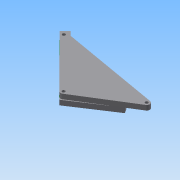
# Autodesk Inventor part: 1-4
Saved by Autodesk Inventor 2015 (Build 190159000, 159)
## iProperties
Created: 2018-05-07
Part Number: 1-4
Material: 一般
Document SubType Name: Modeling
Designer: 王博聖
Density: 1 g/cm^3
Appearance: 預設
Author: 王博聖
Autodesk Inventor part; units mm, degrees
ref_plane "YZ Plane" through (0, 0, 0) normal (1, 0, 0) x (0, 1, 0)
ref_plane "XZ Plane" through (0, 0, 0) normal (0, 1, 0) x (-1, 0, 0)
sketch "草圖1" plane through (0, 0, 0) normal (0, 0, 1) x (1, 0, 0)
  line L0 (0, 0) -> (-20.3496, 20.4644)
  line L1 (-20.3496, 20.4644) -> (21.2832, 13.2109)
  line L2 (21.2832, 13.2109) -> (0, 0)
  line L3 (0, 0) -> (-20.3496, 20.4644) construction
  line L4 (0.8864, 0.8814) -> (-19.4632, 21.3458)
  line L5 (-21.236, 19.583) -> (-0.8864, -0.8814)
  arc A0 (-0.8864, -0.8814) -> (0.8864, 0.8814) centre (0, 0) ccw
  arc A1 (-19.4632, 21.3458) -> (-21.236, 19.583) centre (-20.3496, 20.4644) ccw
  line L6 (-20.3496, 20.4644) -> (21.2832, 13.2109) construction
  line L7 (-20.5642, 19.233) -> (21.0687, 11.9794)
  line L8 (21.4978, 14.4423) -> (-20.1351, 21.6959)
  arc A2 (-20.1351, 21.6959) -> (-20.5642, 19.233) centre (-20.3496, 20.4644) ccw
  arc A3 (21.0687, 11.9794) -> (21.4978, 14.4423) centre (21.2832, 13.2109) ccw
  line L9 (21.2832, 13.2109) -> (0, 0) construction
  line L10 (20.624, 14.2729) -> (-0.6592, 1.062)
  line L11 (0.6592, -1.062) -> (21.9425, 12.1488)
  arc A4 (21.9425, 12.1488) -> (20.624, 14.2729) centre (21.2832, 13.2109) ccw
  arc A5 (-0.6592, 1.062) -> (0.6592, -1.062) centre (0, 0) ccw
  point P0 (-10.1748, 10.2322)
  point P1 (0.4668, 16.8376)
  point P2 (10.6416, 6.6054)
  dimension "d0" = 28.86
  dimension "d1" = 42.26
  dimension "d2" = 25.05
  dimension "d3" = 2.5
  dimension "d4" = 2.5
  dimension "d5" = 2.5
  constraints: 30 end point, 12 point on circle, 12 tangent, 6 centre point, 4 equal length, 3 midpoint, 1 concentric
  measures "d0" distance of L0.start L0.end
  measures "d1" distance of L0.end L1.end
  measures "d2" distance of L1.end L0.start
  measures "d3" diameter of A1
  measures "d4" diameter of A3
  measures "d5" diameter of A5
extrude "擠出1" add sketch "草圖1" along normal blind 2 contours L2 A0 A5 L0 | L0 A5 L10 L4 A0 L2 | A5 L5 A2 L7 L0 | L0 L7 L4 L10 A5 | A0 L4 L10 L7 L2 | L2 L7 A3 L11 A0 | L7 A2 A1 L4 L1 L0 | L0 L1 L4 L7 | L7 L10 L1 L2 | L2 L1 L10 A4 A3 L7 | L4 L1 L10 L7 | L4 A1 L8 A4 L10 L1
sketch "草圖2" plane through (0, 0, 2) normal (0, 0, 1) x (1, 0, 0)
  arc A0 (21.9425, 12.1488) -> (21.4978, 14.4423) centre (21.2832, 13.2109) ccw construction
  arc A1 (-20.1351, 21.6959) -> (-21.236, 19.583) centre (-20.3496, 20.4644) ccw construction
  arc A2 (-0.8864, -0.8814) -> (0.6592, -1.062) centre (0, 0) ccw construction
  circle A3 centre (0, 0) radius 0.625
  circle A4 centre (21.2832, 13.2109) radius 0.625
  circle A5 centre (-20.3496, 20.4644) radius 0.625
  dimension "d8" = 1.25
  dimension "d9" = 1.25
  dimension "d10" = 1.25
  constraints: 3 centre point, 3 coincident
  measures "d8" diameter of A3
  measures "d9" diameter of A4
  measures "d10" diameter of A5
extrude "擠出2" cut sketch "草圖2" against normal blind 2
sketch "草圖3" plane through (0, 0, 0) normal (0, 0, -1) x (-1, 0, 0)
  circle A0 centre (20.3496, 20.4644) radius 0.625 projected
  line L0 (21.236, 19.583) -> (0.8864, -0.8814) projected
  arc A1 (21.236, 19.583) -> (20.1351, 21.6959) centre (20.3496, 20.4644) ccw projected
  line L1 (-21.4978, 14.4423) -> (20.1351, 21.6959) projected
  line L2 (-9.4658, 16.5386) -> (7.2751, 5.5434)
  constraints: 2 end point, 2 point on line
extrude "擠出3" add sketch "草圖3" along normal blind 8
extrude "擠出4" cut sketch "草圖3" along normal blind 6
sketch "草圖4" plane through (-7.2751, 5.5434, -8) normal (0.5489701, -0.835842, 0) x (0.835842, 0.5489701, 0)
  line L0 (20.0288, 0) -> (0, 0)
  line L1 (0, 0) -> (0, 8)
  line L2 (0, 8) -> (20.0288, 8)
  line L3 (20.0288, 8) -> (20.0288, 0)
  point P0 (3.0377, 8)
  constraints: 8 end point, 2 parallel, 1 horizontal, 1 perpendicular
extrude "擠出5" add sketch "草圖4" along normal blind 2
sketch "草圖5" plane through (-7.2751, 5.5434, -8) normal (-0.5489701, 0.835842, 0) x (0.835842, 0.5489701, 0)
  line L0 (0, -8) -> (0, -2) projected
  line L1 (8, -2) -> (-8, -2)
  line L2 (-8, -2) -> (-8, -8)
  line L3 (-8, -8) -> (8, -8)
  line L4 (8, -8) -> (8, -2)
  line L5 (8, -2) -> (-8, -8) construction
  line L6 (-8, -2) -> (8, -8) construction
  point P0 (3.0377, -8)
  point P1 (0, -5)
  dimension "d19" = 16
  dimension "d20" = 6
  constraints: 12 end point, 3 midpoint, 2 parallel, 1 horizontal, 1 perpendicular
  measures "d19" distance of L3.end L2.end
  measures "d20" distance of L2.end L1.end
extrude "擠出6" cut sketch "草圖5" against normal blind 2
sketch "草圖6" plane through (-5.8358, 4.0959, 0) normal (0, 0, 1) x (0.7090931, 0.7051148, 0)
  line L0 (0, 2.0413) -> (0, 0) projected
  line L1 (0, 2.0413) -> (-0.4002, 0.0817) projected
  line L2 (0, 0) -> (-0.4002, 0.0817) projected
  point P0 (1.25, -7.0193)
extrude "擠出7" cut sketch "草圖6" against normal blind 200
sketch "草圖7" plane through (0, 0, 2) normal (0, 0, 1) x (1, 0, 0)
  line L0 (0.1854, 1.5863) -> (-16.6913, 18.5582) projected
  line L1 (-16.6913, 18.5582) -> (17.8364, 12.5426) projected
  line L2 (17.8364, 12.5426) -> (0.1854, 1.5863) projected
extrude "擠出8" add sketch "草圖7" against normal blind 2
sketch "草圖8" plane through (0, 0, 2) normal (0, 0, 1) x (1, 0, 0)
  circle A0 centre (-20.3496, 20.4644) radius 0.625 projected
  line L0 (0.6592, -1.062) -> (21.9425, 12.1488) projected
  arc A1 (21.9425, 12.1488) -> (21.4978, 14.4423) centre (21.2832, 13.2109) ccw projected
  line L1 (21.4978, 14.4423) -> (-20.1351, 21.6959) projected
  arc A2 (-20.1351, 21.6959) -> (-21.236, 19.583) centre (-20.3496, 20.4644) ccw projected
  line L2 (-21.236, 19.583) -> (-0.8864, -0.8814) projected
  arc A3 (-0.8864, -0.8814) -> (0.6592, -1.062) centre (0, 0) ccw projected
  line L3 (9.2581, 16.5748) -> (-33.4865, 24.0221) construction
  line L4 (-20.1351, 21.6959) -> (9.4658, 16.5386) projected
  line L5 (-0.8864, -0.8814) -> (-29.2292, 27.6214)
  line L6 (-29.2292, 27.6214) -> (-26.4102, 29.3712)
  line L7 (-26.4102, 29.3712) -> (-18.4936, 21.4099)
  line L8 (-18.4936, 21.4099) -> (-19.6568, 21.0961)
  line L9 (-19.6568, 21.0961) -> (-20.6706, 21.4099)
  line L10 (-20.6706, 21.4099) -> (-20.8455, 20.8449)
  line L11 (-20.9737, 20.4306) -> (-21.236, 19.583)
  constraints: 16 end point, 2 perpendicular, 2 point on circle, 2 point on line, 1 collinear
extrude "擠出9" add sketch "草圖8" against normal blind 2 contours L5 L6 L7 L1 A2
ref_plane "工作平面1" through (0, 0, -3) normal (0, 0, 1) x (1, 0, 0)
mirror "鏡射1" about plane through (0, 0, -3) normal (0, 0, 1) of "擠出9"
sketch "草圖9" plane through (-7.2751, 5.5434, -8) normal (-0.5489701, 0.835842, 0) x (0.835842, 0.5489701, 0)
  line L0 (8, -2) -> (8, -8) projected
  line L1 (8, -8) -> (20.0288, -8) projected
  line L2 (8, -2) -> (15.2372, -2)
  line L3 (15.2372, -2) -> (15.2372, -8)
  line L4 (15.2372, -8) -> (8, -8)
  line L5 (8, -8) -> (8, -2)
  point P0 (3.0377, -8)
  constraints: 8 end point, 2 parallel, 1 horizontal, 1 perpendicular, 1 point on line
extrude "擠出10" cut sketch "草圖9" against normal blind 10
sketch "草圖10" plane through (-5.8358, 4.0959, -8) normal (-0.7090931, -0.7051148, 0) x (0, 0, 1)
  line L0 (2, 33.1768) -> (8.1848, 33.1768)
  line L1 (5.0924, 33.1768) -> (5.0924, 35.6004)
  circle A0 centre (5.0924, 35.6004) radius 12.9811
  constraints: 4 end point, 1 centre point, 1 coincident, 1 horizontal, 1 midpoint, 1 vertical
extrude "擠出11" cut sketch "草圖10" against normal blind 10
